Autodesk Inventor part; units mm, degrees
(part 8 of 9)
sketch "Sketch44" plane through (0, 0, 0) normal (1, 0, 0) x (0, 0, -1)
  arc A0 (-103.9823, -66.1369) -> (-104.5644, -66.2812) centre (-76.4174, -178.6042) ccw
  arc A1 (-99.4294, -84.7133) -> (-103.9823, -66.1369) centre (-101.7058, -75.4251) ccw
  arc A2 (-99.4294, -84.7133) -> (-99.9153, -84.8337) centre (-76.4174, -178.6042) ccw
  arc A3 (-104.5644, -66.2812) -> (-99.9153, -84.8337) centre (-102.2399, -75.5574) ccw
  arc A4 (-82.1853, 16.259) -> (-85.3603, 13.084) centre (-82.1853, 13.084) ccw
  line L0 (-85.3603, 13.084) -> (-85.3603, 6.734)
  arc A5 (-90.1228, 1.9715) -> (-85.3603, 6.734) centre (-90.1228, 6.734) ccw
  line L1 (-90.1228, 1.9715) -> (-121.8728, 1.9715)
  arc A6 (-126.6353, 6.734) -> (-121.8728, 1.9715) centre (-121.8728, 6.734) ccw
  line L2 (-126.6353, 6.734) -> (-126.6353, 13.084)
  arc A7 (-126.6353, 13.084) -> (-129.8103, 16.259) centre (-129.8103, 13.084) ccw
  line L3 (-129.8103, 16.259) -> (-132.3503, 16.259)
  arc A8 (-132.3503, 22.609) -> (-132.3503, 16.259) centre (-132.3503, 19.434) ccw
  line L4 (-132.3503, 22.609) -> (-129.8103, 22.609)
  arc A9 (-129.8103, 22.609) -> (-126.6353, 25.784) centre (-129.8103, 25.784) ccw
  line L5 (-126.6353, 25.784) -> (-126.6353, 32.134)
  arc A10 (-121.8728, 36.8965) -> (-126.6353, 32.134) centre (-121.8728, 32.134) ccw
  line L6 (-121.8728, 36.8965) -> (-90.1228, 36.8965)
  arc A11 (-85.3603, 32.134) -> (-90.1228, 36.8965) centre (-90.1228, 32.134) ccw
  line L7 (-85.3603, 32.134) -> (-85.3603, 25.784)
  arc A12 (-85.3603, 25.784) -> (-82.1853, 22.609) centre (-82.1853, 25.784) ccw
  line L8 (-82.1853, 22.609) -> (-79.6453, 22.609)
  arc A13 (-79.6453, 16.259) -> (-79.6453, 22.609) centre (-79.6453, 19.434) ccw
  line L9 (-79.6453, 16.259) -> (-82.1853, 16.259)
  line L10 (-112.3478, -13.7765) -> (-99.6478, -13.7765)
  arc A14 (-99.6478, -18.8819) -> (-99.6478, -13.7765) centre (-99.6478, -16.3292) ccw
  line L11 (-99.6478, -18.8819) -> (-112.3478, -18.8819)
  arc A15 (-112.3478, -13.7765) -> (-112.3478, -18.8819) centre (-112.3478, -16.3292) ccw
  circle A16 centre (-58.8554, 19.434) radius 2.4892
  line L12 (-177.4857, -133.2108) -> (-177.0061, -133.3781)
  arc A17 (-183.3071, -151.4366) -> (-177.0061, -133.3781) centre (-180.1566, -142.4074) ccw
  line L13 (-183.3071, -151.4366) -> (-183.7867, -151.2692)
  arc A18 (-177.4857, -133.2108) -> (-183.7867, -151.2692) centre (-180.6362, -142.24) ccw
  circle A19 centre (-76.4174, -178.6042) radius 13.335
  circle A20 centre (-187.1176, -166.8269) radius 2.4892
  circle A21 centre (-174.2102, -166.8866) radius 2.4892
  circle A22 centre (-167.2175, -120.5501) radius 2.4892
  circle A23 centre (-180.1195, -116.9252) radius 2.4892
  circle A24 centre (-193.0957, -120.1058) radius 2.4892
  circle A25 centre (-186.8225, -117.6771) radius 2.4892
  circle A26 centre (-173.4354, -117.9041) radius 2.4892
  circle A27 centre (-168.1768, -164.3742) radius 2.4892
  circle A28 centre (-180.6733, -167.7222) radius 2.4892
  circle A29 centre (-193.0957, -164.2646) radius 2.4892
  circle A30 centre (-85.7798, -94.9817) radius 2.4892
  circle A31 centre (-110.3931, -99.2933) radius 2.4892
  circle A32 centre (-101.8395, -50.0579) radius 2.4892
  circle A33 centre (-124.2369, -62.8574) radius 2.4892
  circle A34 centre (-110.6604, -51.6228) radius 2.4892
  circle A35 centre (-93.2858, -99.3592) radius 2.4892
  circle A36 centre (-118.4334, -56.0666) radius 2.4892
  circle A37 centre (-93.0185, -51.5569) radius 2.4892
  circle A38 centre (-101.8395, -100.8579) radius 2.4892
  circle A39 centre (-80.2428, -88.2574) radius 2.4892
  circle A40 centre (239.2356, -31.496) radius 3.3782
  circle A41 centre (223.7295, 90.3926) radius 3.3782
  circle A42 centre (239.2356, 31.496) radius 3.3782
  circle A43 centre (192.7107, -145.218) radius 3.3782
  line L14 (149.831, -89.2272) -> (89.9434, -38.9755)
  arc A44 (88.9, -36.7379) -> (89.9434, -38.9755) centre (91.821, -36.7379) ccw
  line L15 (88.9, -36.7379) -> (88.9, -15.621)
  arc A45 (91.821, -12.7) -> (88.9, -15.621) centre (91.821, -15.621) ccw
  line L16 (91.821, -12.7) -> (174.1799, -12.7)
  arc A46 (177.0893, -15.8819) -> (174.1799, -12.7) centre (174.1799, -15.621) ccw
  arc A47 (154.2425, -88.4425) -> (177.0893, -15.8819) centre (0, 0) ccw
  arc A48 (149.831, -89.2272) -> (154.2425, -88.4425) centre (151.7086, -86.9895) ccw
  line L17 (88.9, -0.254) -> (88.9, 0.254)
  arc A49 (91.821, 3.175) -> (88.9, 0.254) centre (91.821, 0.254) ccw
  line L18 (91.821, 3.175) -> (174.4218, 3.175)
  arc A50 (177.3428, 0.254) -> (174.4218, 3.175) centre (174.4218, 0.254) ccw
  line L19 (177.3428, 0.254) -> (177.3428, -0.254)
  arc A51 (174.4218, -3.175) -> (177.3428, -0.254) centre (174.4218, -0.254) ccw
  line L20 (174.4218, -3.175) -> (91.821, -3.175)
  arc A52 (88.9, -0.254) -> (91.821, -3.175) centre (91.821, -0.254) ccw
  arc A53 (177.0893, 15.8819) -> (169.6939, 53.0738) centre (0, 0) ccw
  arc A54 (174.1799, 12.7) -> (177.0893, 15.8819) centre (174.1799, 15.621) ccw
  line L21 (174.1799, 12.7) -> (91.821, 12.7)
  arc A55 (88.9, 15.621) -> (91.821, 12.7) centre (91.821, 15.621) ccw
  line L22 (88.9, 15.621) -> (88.9, 17.1891)
  arc A56 (90.5865, 19.8364) -> (88.9, 17.1891) centre (91.821, 17.1891) ccw
  line L23 (90.5865, 19.8364) -> (165.6716, 54.8492)
  arc A57 (169.6939, 53.0738) -> (165.6716, 54.8492) centre (166.9061, 52.2019) ccw
  arc A58 (180.8991, -105.7674) -> (203.0448, 51.8076) centre (0, 0) ccw
  arc A59 (204.8485, 54.889) -> (203.0448, 51.8076) centre (205.5059, 52.4355) ccw
  line L24 (204.8485, 54.889) -> (206.0753, 55.2177)
  arc A60 (209.1938, 53.3924) -> (206.0753, 55.2177) centre (206.7327, 52.7643) ccw
  arc A61 (186.3731, -108.9857) -> (209.1938, 53.3924) centre (0, 0) ccw
  arc A62 (182.8723, -109.8807) -> (186.3731, -108.9857) centre (184.1805, -107.7035) ccw
  line L25 (182.8723, -109.8807) -> (181.7836, -109.2266)
  arc A63 (180.8991, -105.7674) -> (181.7836, -109.2266) centre (183.0918, -107.0494) ccw
  arc A64 (159.1231, -92.6879) -> (178.5072, 45.237) centre (0, 0) ccw
  arc A65 (180.312, 48.3145) -> (178.5072, 45.237) centre (180.9694, 45.861) ccw
  line L26 (180.312, 48.3145) -> (181.5388, 48.6432)
  arc A66 (184.6584, 46.8139) -> (181.5388, 48.6432) centre (182.1962, 46.1897) ccw
  arc A67 (164.6013, -95.8992) -> (184.6584, 46.8139) centre (0, 0) ccw
  arc A68 (161.0985, -96.7977) -> (164.6013, -95.8992) centre (162.4067, -94.6205) ccw
  line L27 (161.0985, -96.7977) -> (160.0098, -96.1436)
  arc A69 (159.1231, -92.6879) -> (160.0098, -96.1436) centre (161.3179, -93.9664) ccw
  line L28 (171.9854, -103.3393) -> (170.8967, -102.6851)
  arc A70 (170.0112, -99.2275) -> (170.8967, -102.6851) centre (172.2049, -100.5079) ccw
  arc A71 (170.0112, -99.2275) -> (190.7761, 48.5222) centre (0, 0) ccw
  arc A72 (192.5803, 51.6017) -> (190.7761, 48.5222) centre (193.2377, 49.1483) ccw
  line L29 (192.5803, 51.6017) -> (193.8071, 51.9305)
  arc A73 (196.9261, 50.1033) -> (193.8071, 51.9305) centre (194.4645, 49.477) ccw
  arc A74 (175.4872, -102.4426) -> (196.9261, 50.1033) centre (0, 0) ccw
  arc A75 (171.9854, -103.3393) -> (175.4872, -102.4426) centre (173.2936, -101.1621) ccw
  circle A76 centre (187.962, 68.4126) radius 2.5527
  circle A77 centre (0, 0) radius 13.335
  circle A78 centre (160.7915, -118.9794) radius 2.5527
  circle A79 centre (145.0649, -113.4346) radius 2.5527
  circle A80 centre (122.2368, -242.899) radius 2.5527
  circle A81 centre (70.3186, -242.899) radius 2.5527
  circle A82 centre (97.9437, -242.899) radius 2.5527
  circle A83 centre (145.0649, -242.899) radius 2.5527
  circle A84 centre (-116.932, -242.899) radius 2.5527
  circle A85 centre (-116.932, -179.399) radius 2.5527
  circle A86 centre (-148.682, -179.399) radius 2.5527
  circle A87 centre (-186.782, -39.699) radius 2.5527
  circle A88 centre (-186.782, -242.899) radius 2.5527
  circle A89 centre (67.218, 63.5) radius 2.5527
  circle A90 centre (-59.782, 63.5) radius 2.5527
  circle A91 centre (-8.982, 63.5) radius 2.5527
  circle A92 centre (143.418, 63.5) radius 2.5527
  circle A93 centre (-186.782, -179.399) radius 2.5527
  circle A94 centre (-148.682, -39.699) radius 2.5527
  circle A95 centre (-116.932, -39.699) radius 2.5527
  circle A96 centre (-148.682, -242.899) radius 2.5527
  circle A97 centre (11.1125, -19.2474) radius 2.2479
  circle A98 centre (-22.225, 0) radius 2.2479
  circle A99 centre (11.1125, 19.2474) radius 2.2479
  circle A100 centre (22.225, 0) radius 2.2479
  circle A101 centre (-11.1125, 19.2474) radius 2.2479
  circle A102 centre (-11.1125, -19.2474) radius 2.2479
  line L30 (-80.5978, 54.7781) -> (-131.3978, 54.7781)
  arc A103 (-131.3978, 59.8835) -> (-131.3978, 54.7781) centre (-131.3978, 57.3308) ccw
  line L31 (-131.3978, 59.8835) -> (-80.5978, 59.8835)
  arc A104 (-80.5978, 54.7781) -> (-80.5978, 59.8835) centre (-80.5978, 57.3308) ccw
  circle A105 centre (-123.52, 44.45) radius 2.4892
  arc A106 (-166.8187, -7.1514) -> (-170.0188, -10.965) centre (-168.4187, -9.0582) ccw
  arc A107 (-166.8187, -7.1514) -> (-135.2171, -21.8874) centre (-123.52, 44.45) ccw
  arc A108 (-136.0816, -26.7902) -> (-135.2171, -21.8874) centre (-135.6494, -24.3388) ccw
  arc A109 (-170.0188, -10.965) -> (-136.0816, -26.7902) centre (-123.52, 44.45) ccw
  arc A110 (-196.307, 76.2) -> (-199.482, 73.025) centre (-196.307, 73.025) ccw
  line L32 (-199.482, 73.025) -> (-199.482, -252.424)
  arc A111 (-199.482, -252.424) -> (-196.307, -255.599) centre (-196.307, -252.424) ccw
  line L33 (-196.307, -255.599) -> (147.8383, -255.599)
  arc A112 (147.8383, -255.599) -> (150.6952, -253.8092) centre (147.8383, -252.424) ccw
  line L34 (194.4526, -163.563) -> (150.6952, -253.8092)
  arc A113 (194.8736, -162.9119) -> (194.4526, -163.563) centre (197.3095, -164.9483) ccw
  arc A114 (194.8736, -162.9119) -> (235.5329, 95.0804) centre (0, 0) ccw
  arc A115 (235.5329, 95.0804) -> (218.389, 101.8364) centre (223.7562, 90.3263) ccw
  line L35 (218.389, 101.8364) -> (173.6183, 80.9596)
  arc A116 (152.1493, 76.2) -> (173.6183, 80.9596) centre (152.1493, 127) ccw
  line L36 (152.1493, 76.2) -> (-196.307, 76.2)
  arc A117 (-85.6539, -48.4094) -> (-88.99, -46.6745) centre (-90.1204, -52.923) ccw
  arc A118 (-114.689, -104.2414) -> (-85.6539, -48.4094) centre (-101.8395, -75.4579) ccw
  arc A119 (-118.0252, -102.5065) -> (-114.689, -104.2414) centre (-113.5587, -97.9928) ccw
  arc A120 (-88.99, -46.6745) -> (-118.0252, -102.5065) centre (-101.8395, -75.4579) ccw
  arc A121 (-84.1306, -35.1868) -> (-84.8012, -35.3982) centre (-84.3454, -35.6751) ccw
  arc A122 (-85.259, -35.965) -> (-84.8012, -35.3982) centre (-87.1419, -33.9761) ccw
  arc A123 (-87.6678, -35.0381) -> (-85.259, -35.965) centre (-86.2421, -34.9266) ccw
  arc A124 (-87.6275, -34.3106) -> (-87.6678, -35.0381) centre (-84.9373, -34.8245) ccw
  arc A125 (-87.6275, -34.3106) -> (-87.9834, -33.7042) centre (-88.1514, -34.2105) ccw
  arc A126 (-87.9834, -33.7042) -> (-88.7509, -33.4573) centre (-101.8395, -75.4579) ccw
  arc A127 (-88.7509, -33.4573) -> (-89.3936, -33.7424) centre (-88.9096, -33.9665) ccw
  arc A128 (-89.7851, -34.3569) -> (-89.3936, -33.7424) centre (-91.8788, -32.5913) ccw
  arc A129 (-92.2825, -33.7055) -> (-89.7851, -34.3569) centre (-90.8783, -33.4351) ccw
  arc A130 (-92.3239, -32.978) -> (-92.2825, -33.7055) centre (-89.5931, -33.1875) ccw
  arc A131 (-92.3239, -32.978) -> (-92.7455, -32.4154) centre (-92.8557, -32.9372) ccw
  arc A132 (-92.7455, -32.4154) -> (-93.5358, -32.2559) centre (-101.8395, -75.4579) ccw
  arc A133 (-93.5358, -32.2559) -> (-94.1425, -32.6112) centre (-93.6365, -32.7797) ccw
  arc A134 (-94.4627, -33.2657) -> (-94.1425, -32.6112) centre (-96.741, -31.7456) ccw
  arc A135 (-97.0174, -32.898) -> (-94.4627, -33.2657) centre (-95.6523, -32.472) ccw
  arc A136 (-97.14, -32.1797) -> (-97.0174, -32.898) centre (-94.4029, -32.0822) ccw
  arc A137 (-97.14, -32.1797) -> (-97.6219, -31.6678) centre (-97.673, -32.1987) ccw
  arc A138 (-97.6219, -31.6678) -> (-98.4251, -31.5978) centre (-101.8395, -75.4579) ccw
  arc A139 (-98.4251, -31.5978) -> (-98.9883, -32.0188) centre (-98.4665, -32.1296) ccw
  arc A140 (-99.2331, -32.7051) -> (-98.9883, -32.0188) centre (-101.6673, -31.4496) ccw
  arc A141 (-101.8129, -32.6257) -> (-99.2331, -32.7051) centre (-100.5041, -32.0496) ccw
  arc A142 (-102.0151, -31.9257) -> (-101.8129, -32.6257) centre (-99.3062, -31.5223) ccw
  arc A143 (-102.0151, -31.9257) -> (-102.5514, -31.4709) centre (-102.5427, -32.0042) ccw
  arc A144 (-102.5514, -31.4709) -> (-103.3573, -31.4913) centre (-101.8395, -75.4579) ccw
  arc A145 (-103.3573, -31.4913) -> (-103.8698, -31.9727) centre (-103.3389, -32.0244) ccw
  arc A146 (-104.0363, -32.6821) -> (-103.8698, -31.9727) centre (-106.5957, -31.7071) ccw
  arc A147 (-106.6088, -32.892) -> (-104.0363, -32.6821) centre (-105.3727, -32.173) ccw
  arc A148 (-106.8881, -32.2191) -> (-106.6088, -32.892) centre (-104.2414, -31.5149) ccw
  arc A149 (-106.8881, -32.2191) -> (-107.4719, -31.8272) centre (-107.4036, -32.3562) ccw
  arc A150 (-107.4719, -31.8272) -> (-108.2705, -31.9377) centre (-101.8395, -75.4579) ccw
  arc A151 (-108.2705, -31.9377) -> (-108.7259, -32.4734) centre (-108.1925, -32.4654) ccw
  arc A152 (-108.8119, -33.197) -> (-108.7259, -32.4734) centre (-111.4644, -32.5147) ccw
  arc A153 (-111.3446, -33.6937) -> (-108.8119, -33.197) centre (-110.1968, -32.8407) ccw
  arc A154 (-111.6976, -33.0562) -> (-111.3446, -33.6937) centre (-109.1463, -32.0601) ccw
  arc A155 (-111.6976, -33.0562) -> (-112.3216, -32.7321) centre (-112.1945, -33.2502) ccw
  arc A156 (-112.3216, -32.7321) -> (-113.1028, -32.9314) centre (-101.8395, -75.4579) ccw
  arc A157 (-113.1028, -32.9314) -> (-113.4953, -33.5147) centre (-112.9662, -33.447) ccw
  arc A158 (-113.4998, -34.2434) -> (-113.4953, -33.5147) centre (-116.212, -33.8623) ccw
  arc A159 (-115.961, -35.0205) -> (-113.4998, -34.2434) centre (-114.9159, -34.0444) ccw
  arc A160 (-116.3831, -34.4266) -> (-115.961, -35.0205) centre (-113.9594, -33.1511) ccw
  arc A161 (-116.3831, -34.4266) -> (-117.0394, -34.1744) centre (-116.8551, -34.675) ccw
  arc A162 (-117.0394, -34.1744) -> (-117.7934, -34.4599) centre (-101.8395, -75.4579) ccw
  arc A163 (-117.7934, -34.4599) -> (-118.1182, -35.0835) centre (-117.6, -34.957) ccw
  arc A164 (-118.041, -35.8081) -> (-118.1182, -35.0835) centre (-120.7788, -35.7331) ccw
  arc A165 (-120.3998, -36.8559) -> (-118.041, -35.8081) centre (-119.4705, -35.7689) ccw
  arc A166 (-120.8857, -36.3129) -> (-120.3998, -36.8559) centre (-118.6201, -34.7741) ccw
  arc A167 (-120.8857, -36.3129) -> (-121.5661, -36.1358) centre (-121.327, -36.6126) ccw
  arc A168 (-121.5661, -36.1358) -> (-122.2834, -36.5039) centre (-101.8395, -75.4579) ccw
  arc A169 (-122.2834, -36.5039) -> (-122.5363, -37.16) centre (-122.0356, -36.9763) ccw
  arc A170 (-122.3785, -37.8714) -> (-122.5363, -37.16) centre (-125.1075, -38.1034) ccw
  arc A171 (-124.6051, -39.1767) -> (-122.3785, -37.8714) centre (-123.8034, -37.9925) ccw
  arc A172 (-125.1488, -38.6915) -> (-124.6051, -39.1767) centre (-123.0697, -36.9087) ccw
  arc A173 (-125.1488, -38.6915) -> (-125.8448, -38.5918) centre (-125.5537, -39.0388) ccw
  arc A174 (-125.8448, -38.5918) -> (-126.5163, -39.0379) centre (-101.8395, -75.4579) ccw
  arc A175 (-126.5163, -39.0379) -> (-126.6942, -39.7181) centre (-126.2171, -39.4795) ccw
  arc A176 (-126.4578, -40.4073) -> (-126.6942, -39.7181) centre (-129.1436, -40.9435) ccw
  arc A177 (-128.5242, -41.9537) -> (-126.4578, -40.4073) centre (-127.8601, -40.6873) ccw
  arc A178 (-129.1188, -41.5325) -> (-128.5242, -41.9537) centre (-127.2523, -39.5281) ccw
  arc A179 (-129.1188, -41.5325) -> (-129.8215, -41.5113) centre (-129.4823, -41.9229) ccw
  arc A180 (-129.8215, -41.5113) -> (-130.4389, -42.0298) centre (-101.8395, -75.4579) ccw
  arc A181 (-130.4389, -42.0298) -> (-130.5395, -42.7257) centre (-130.0922, -42.4351) ccw
  arc A182 (-130.2274, -43.3841) -> (-130.5395, -42.7257) centre (-132.8363, -44.2176) ccw
  arc A183 (-132.1077, -45.1521) -> (-130.2274, -43.3841) centre (-131.5896, -43.8193) ccw
  arc A184 (-132.7457, -44.8002) -> (-132.1077, -45.1521) centre (-131.1154, -42.5994) ccw
  arc A185 (-132.7457, -44.8002) -> (-133.4464, -44.8577) centre (-133.0632, -45.2288) ccw
  arc A186 (-133.4464, -44.8577) -> (-134.0019, -45.4421) centre (-101.8395, -75.4579) ccw
  arc A187 (-134.0019, -45.4421) -> (-134.0239, -46.1449) centre (-133.6119, -45.806) ccw
  arc A188 (-133.64, -46.7642) -> (-134.0239, -46.1449) centre (-136.1392, -47.8845) ccw
  arc A189 (-135.3105, -48.7317) -> (-133.64, -46.7642) centre (-134.9449, -47.3492) ccw
  arc A190 (-135.9839, -48.4533) -> (-135.3105, -48.7317) centre (-134.6103, -46.0839) ccw
  arc A191 (-135.9839, -48.4533) -> (-136.6738, -48.589) centre (-136.2514, -48.9148) ccw
  arc A192 (-136.6738, -48.589) -> (-137.1604, -49.2319) centre (-101.8395, -75.4579) ccw
  arc A193 (-137.1604, -49.2319) -> (-137.1035, -49.9327) centre (-136.7321, -49.5499) ccw
  arc A194 (-136.6528, -50.5051) -> (-137.1035, -49.9327) centre (-139.0108, -51.8983) ccw
  arc A195 (-138.0925, -52.6473) -> (-136.6528, -50.5051) centre (-137.884, -51.2325) ccw
  arc A196 (-138.7928, -52.4461) -> (-138.0925, -52.6473) centre (-137.6931, -49.9377) ccw
  arc A197 (-138.7928, -52.4461) -> (-139.4631, -52.6581) centre (-139.007, -52.9346) ccw
  arc A198 (-139.4631, -52.6581) -> (-139.8746, -53.3515) centre (-101.8395, -75.4579) ccw
  arc A199 (-139.8746, -53.3515) -> (-139.7397, -54.0415) centre (-139.4135, -53.6195) ccw
  arc A200 (-139.2277, -54.5599) -> (-139.7397, -54.0415) centre (-141.4149, -56.2083) ccw
  arc A201 (-140.4185, -56.8497) -> (-139.2277, -54.5599) centre (-140.3697, -55.4205) ccw
  arc A202 (-141.137, -56.7282) -> (-140.4185, -56.8497) centre (-140.325, -54.1125) ccw
  arc A203 (-141.137, -56.7282) -> (-141.7793, -57.014) centre (-141.2951, -57.2376) ccw
  arc A204 (-141.7793, -57.014) -> (-142.1106, -57.749) centre (-101.8395, -75.4579) ccw
  arc A205 (-142.1106, -57.749) -> (-141.8993, -58.4196) centre (-141.6224, -57.9638) ccw
  arc A206 (-141.3324, -58.8774) -> (-141.8993, -58.4196) centre (-143.3214, -60.7603) ccw
  arc A207 (-142.2594, -61.2862) -> (-141.3324, -58.8774) centre (-142.3709, -59.8605) ccw
  arc A208 (-142.9869, -61.2459) -> (-142.2594, -61.2862) centre (-142.473, -58.5557) ccw
  arc A209 (-142.9869, -61.2459) -> (-143.5933, -61.6018) centre (-143.087, -61.7698) ccw
  arc A210 (-143.5933, -61.6018) -> (-143.8402, -62.3693) centre (-101.8395, -75.4579) ccw
  arc A211 (-143.8402, -62.3693) -> (-143.5551, -63.012) centre (-143.3309, -62.528) ccw
  arc A212 (-142.9405, -63.4035) -> (-143.5551, -63.012) centre (-144.7061, -65.4972) ccw
  arc A213 (-143.592, -65.9009) -> (-142.9405, -63.4035) centre (-143.8624, -64.4967) ccw
  arc A214 (-144.3194, -65.9423) -> (-143.592, -65.9009) centre (-144.1099, -63.2115) ccw
  arc A215 (-144.3194, -65.9423) -> (-144.8821, -66.3639) centre (-144.3602, -66.4741) ccw
  arc A216 (-144.8821, -66.3639) -> (-145.0416, -67.1542) centre (-101.8395, -75.4579) ccw
  arc A217 (-145.0416, -67.1542) -> (-144.6863, -67.7609) centre (-144.5177, -67.2549) ccw
  arc A218 (-144.0318, -68.0811) -> (-144.6863, -67.7609) centre (-145.5519, -70.3594) ccw
  arc A219 (-144.3995, -70.6358) -> (-144.0318, -68.0811) centre (-144.8255, -69.2707) ccw
  arc A220 (-145.1178, -70.7584) -> (-144.3995, -70.6358) centre (-145.2153, -68.0213) ccw
  arc A221 (-145.1178, -70.7584) -> (-145.6297, -71.2403) centre (-145.0988, -71.2914) ccw
  arc A222 (-145.6297, -71.2403) -> (-145.6996, -72.0435) centre (-101.8395, -75.4579) ccw
  arc A223 (-145.6996, -72.0435) -> (-145.2787, -72.6067) centre (-145.1678, -72.0849) ccw
  arc A224 (-144.5924, -72.8515) -> (-145.2787, -72.6067) centre (-145.8479, -75.2857) ccw
  arc A225 (-144.6718, -75.4313) -> (-144.5924, -72.8515) centre (-145.2479, -74.1225) ccw
  arc A226 (-145.3718, -75.6336) -> (-144.6718, -75.4313) centre (-145.7752, -72.9246) ccw
  arc A227 (-145.3718, -75.6336) -> (-145.8266, -76.1698) centre (-145.2932, -76.1611) ccw
  arc A228 (-145.8266, -76.1698) -> (-145.8061, -76.9757) centre (-101.8395, -75.4579) ccw
  arc A229 (-145.8061, -76.9757) -> (-145.3248, -77.4882) centre (-145.2731, -76.9573) ccw
  arc A230 (-144.6154, -77.6547) -> (-145.3248, -77.4882) centre (-145.5904, -80.2141) ccw
  arc A231 (-144.4054, -80.2272) -> (-144.6154, -77.6547) centre (-145.1245, -78.9911) ccw
  arc A232 (-145.0784, -80.5065) -> (-144.4054, -80.2272) centre (-145.7826, -77.8598) ccw
  arc A233 (-145.0784, -80.5065) -> (-145.4703, -81.0903) centre (-144.9413, -81.022) ccw
  arc A234 (-145.4703, -81.0903) -> (-145.3598, -81.8889) centre (-101.8395, -75.4579) ccw
  arc A235 (-145.3598, -81.8889) -> (-144.824, -82.3443) centre (-144.8321, -81.8109) ccw
  arc A236 (-144.1005, -82.4303) -> (-144.824, -82.3443) centre (-144.7828, -85.0828) ccw
  arc A237 (-143.6038, -84.9631) -> (-144.1005, -82.4303) centre (-144.4567, -83.8152) ccw
  arc A238 (-144.2413, -85.316) -> (-143.6038, -84.9631) centre (-145.2374, -82.7647) ccw
  arc A239 (-144.2413, -85.316) -> (-144.5653, -85.94) centre (-144.0473, -85.8129) ccw
  arc A240 (-144.5653, -85.94) -> (-144.3661, -86.7212) centre (-101.8395, -75.4579) ccw
  arc A241 (-144.3661, -86.7212) -> (-143.7827, -87.1137) centre (-143.8504, -86.5846) ccw
  arc A242 (-143.0541, -87.1182) -> (-143.7827, -87.1137) centre (-143.4351, -89.8304) ccw
  arc A243 (-142.277, -89.5794) -> (-143.0541, -87.1182) centre (-143.2531, -88.5343) ccw
  arc A244 (-142.8709, -90.0015) -> (-142.277, -89.5794) centre (-144.1464, -87.5778) ccw
  arc A245 (-142.8709, -90.0015) -> (-143.1231, -90.6578) centre (-142.6225, -90.4735) ccw
  arc A246 (-143.1231, -90.6578) -> (-142.8376, -91.4118) centre (-101.8395, -75.4579) ccw
  arc A247 (-142.8376, -91.4118) -> (-142.214, -91.7366) centre (-142.3405, -91.2184) ccw
  arc A248 (-141.4894, -91.6594) -> (-142.214, -91.7366) centre (-141.5644, -94.3972) ccw
  arc A249 (-140.4416, -94.0182) -> (-141.4894, -91.6594) centre (-141.5286, -93.0889) ccw
  arc A250 (-140.9846, -94.5041) -> (-140.4416, -94.0182) centre (-142.5234, -92.2385) ccw
  arc A251 (-140.9846, -94.5041) -> (-141.1616, -95.1845) centre (-140.6849, -94.9454) ccw
  arc A252 (-141.1616, -95.1845) -> (-140.7935, -95.9018) centre (-101.8395, -75.4579) ccw
  arc A253 (-140.7935, -95.9018) -> (-140.1375, -96.1547) centre (-140.3212, -95.654) ccw
  arc A254 (-139.4261, -95.997) -> (-140.1375, -96.1547) centre (-139.1941, -98.7259) ccw
  arc A255 (-138.1208, -98.2235) -> (-139.4261, -95.997) centre (-139.305, -97.4218) ccw
  arc A256 (-138.6059, -98.7672) -> (-138.1208, -98.2235) centre (-140.3888, -96.6881) ccw
  arc A257 (-138.6059, -98.7672) -> (-138.7057, -99.4632) centre (-138.2587, -99.1721) ccw
  arc A258 (-138.7057, -99.4632) -> (-138.2596, -100.1348) centre (-101.8395, -75.4579) ccw
  arc A259 (-138.2596, -100.1348) -> (-137.5794, -100.3126) centre (-137.818, -99.8356) ccw
  arc A260 (-136.8901, -100.0762) -> (-137.5794, -100.3126) centre (-136.354, -102.762) ccw
  arc A261 (-135.3437, -102.1426) -> (-136.8901, -100.0762) centre (-136.6102, -101.4785) ccw
  arc A262 (-135.7649, -102.7372) -> (-135.3437, -102.1426) centre (-137.7693, -100.8707) ccw
  arc A263 (-135.7649, -102.7372) -> (-135.7862, -103.4399) centre (-135.3746, -103.1007) ccw
  arc A264 (-135.7862, -103.4399) -> (-135.2677, -104.0573) centre (-101.8395, -75.4579) ccw
  arc A265 (-135.2677, -104.0573) -> (-134.5718, -104.1579) centre (-134.8624, -103.7106) ccw
  arc A266 (-133.9134, -103.8458) -> (-134.5718, -104.1579) centre (-133.0799, -106.4547) ccw
  arc A267 (-132.1453, -105.7261) -> (-133.9134, -103.8458) centre (-133.4782, -105.208) ccw
  arc A268 (-132.4973, -106.3641) -> (-132.1453, -105.7261) centre (-134.6981, -104.7338) ccw
  arc A269 (-132.4973, -106.3641) -> (-132.4397, -107.0648) centre (-132.0687, -106.6816) ccw
  arc A270 (-132.4397, -107.0648) -> (-131.8554, -107.6203) centre (-101.8395, -75.4579) ccw
  arc A271 (-131.8554, -107.6203) -> (-131.1526, -107.6423) centre (-131.4914, -107.2303) ccw
  arc A272 (-130.5333, -107.2584) -> (-131.1526, -107.6423) centre (-129.4129, -109.7576) ccw
  arc A273 (-128.5658, -108.9289) -> (-130.5333, -107.2584) centre (-129.9483, -108.5633) ccw
  arc A274 (-128.8442, -109.6023) -> (-128.5658, -108.9289) centre (-131.2136, -108.2287) ccw
  arc A275 (-128.8442, -109.6023) -> (-128.7085, -110.2922) centre (-128.3827, -109.8699) ccw
  arc A276 (-128.7085, -110.2922) -> (-128.0656, -110.7788) centre (-101.8395, -75.4579) ccw
  arc A277 (-128.0656, -110.7788) -> (-127.3648, -110.722) centre (-127.7476, -110.3505) ccw
  arc A278 (-126.7923, -110.2712) -> (-127.3648, -110.722) centre (-125.3992, -112.6292) ccw
  arc A279 (-124.6502, -111.7109) -> (-126.7923, -110.2712) centre (-126.065, -111.5024) ccw
  arc A280 (-124.8514, -112.4112) -> (-124.6502, -111.7109) centre (-127.3598, -111.3115) ccw
  arc A281 (-124.8514, -112.4112) -> (-124.6393, -113.0815) centre (-124.3629, -112.6254) ccw
  arc A282 (-124.6393, -113.0815) -> (-123.946, -113.4931) centre (-101.8395, -75.4579) ccw
  arc A283 (-123.946, -113.4931) -> (-123.256, -113.3581) centre (-123.678, -113.0319) ccw
  arc A284 (-122.7376, -112.8461) -> (-123.256, -113.3581) centre (-121.0892, -115.0333) ccw
  arc A285 (-120.4477, -114.0369) -> (-122.7376, -112.8461) centre (-121.8769, -113.9881) ccw
  arc A286 (-120.5693, -114.7554) -> (-120.4477, -114.0369) centre (-123.185, -113.9434) ccw
  arc A287 (-120.5693, -114.7554) -> (-120.2835, -115.3977) centre (-120.0598, -114.9135) ccw
  arc A288 (-120.2835, -115.3977) -> (-119.5484, -115.729) centre (-101.8395, -75.4579) ccw
  arc A289 (-119.5484, -115.729) -> (-118.8779, -115.5177) centre (-119.3337, -115.2408) ccw
  arc A290 (-118.4201, -114.9508) -> (-118.8779, -115.5177) centre (-116.5372, -116.9398) ccw
  arc A291 (-116.0113, -115.8778) -> (-118.4201, -114.9508) centre (-117.4369, -115.9893) ccw
  arc A292 (-116.0516, -116.6053) -> (-116.0113, -115.8778) centre (-118.7417, -116.0914) ccw
  arc A293 (-116.0516, -116.6053) -> (-115.6957, -117.2117) centre (-115.5277, -116.7054) ccw
  arc A294 (-115.6957, -117.2117) -> (-114.9282, -117.4586) centre (-101.8395, -75.4579) ccw
  arc A295 (-114.9282, -117.4586) -> (-114.2855, -117.1735) centre (-114.7695, -116.9493) ccw
  arc A296 (-113.894, -116.5589) -> (-114.2855, -117.1735) centre (-111.8002, -118.3245) ccw
  arc A297 (-111.3966, -117.2104) -> (-113.894, -116.5589) centre (-112.8008, -117.4808) ccw
  arc A298 (-111.3552, -117.9379) -> (-111.3966, -117.2104) centre (-114.086, -117.7283) ccw
  arc A299 (-111.3552, -117.9379) -> (-110.9336, -118.5005) centre (-110.8233, -117.9787) ccw
  arc A300 (-110.9336, -118.5005) -> (-110.1433, -118.66) centre (-101.8395, -75.4579) ccw
  arc A301 (-110.1433, -118.66) -> (-109.5365, -118.3047) centre (-110.0426, -118.1361) ccw
  arc A302 (-109.2163, -117.6502) -> (-109.5365, -118.3047) centre (-106.9381, -119.1703) ccw
  arc A303 (-106.6617, -118.0179) -> (-109.2163, -117.6502) centre (-108.0268, -118.4439) ccw
  arc A304 (-106.5391, -118.7362) -> (-106.6617, -118.0179) centre (-109.2762, -118.8337) ccw
  arc A305 (-106.5391, -118.7362) -> (-106.0572, -119.2481) centre (-106.006, -118.7172) ccw
  arc A306 (-106.0572, -119.2481) -> (-105.254, -119.318) centre (-101.8395, -75.4579) ccw
  arc A307 (-105.254, -119.318) -> (-104.6908, -118.8971) centre (-105.2126, -118.7862) ccw
  arc A308 (-104.4459, -118.2108) -> (-104.6908, -118.8971) centre (-102.0118, -119.4663) ccw
  arc A309 (-101.8662, -118.2902) -> (-104.4459, -118.2108) centre (-103.175, -118.8663) ccw
  arc A310 (-101.6639, -118.9902) -> (-101.8662, -118.2902) centre (-104.3729, -119.3936) ccw
  arc A311 (-101.6639, -118.9902) -> (-101.1277, -119.445) centre (-101.1363, -118.9117) ccw
  arc A312 (-101.1277, -119.445) -> (-100.3217, -119.4246) centre (-101.8395, -75.4579) ccw
  arc A313 (-100.3217, -119.4246) -> (-99.8092, -118.9432) centre (-100.3401, -118.8915) ccw
  arc A314 (-99.6427, -118.2338) -> (-99.8092, -118.9432) centre (-97.0833, -119.2088) ccw
  arc A315 (-97.0703, -118.0239) -> (-99.6427, -118.2338) centre (-98.3064, -118.7429) ccw
  arc A316 (-96.791, -118.6968) -> (-97.0703, -118.0239) centre (-99.4377, -119.401) ccw
  arc A317 (-96.791, -118.6968) -> (-96.2072, -119.0887) centre (-96.2755, -118.5597) ccw
  arc A318 (-96.2072, -119.0887) -> (-95.4086, -118.9782) centre (-101.8395, -75.4579) ccw
  arc A319 (-95.4086, -118.9782) -> (-94.9532, -118.4425) centre (-95.4866, -118.4505) ccw
  arc A320 (-94.8672, -117.7189) -> (-94.9532, -118.4425) centre (-92.2147, -118.4012) ccw
  arc A321 (-92.3344, -117.2222) -> (-94.8672, -117.7189) centre (-93.4822, -118.0752) ccw
  arc A322 (-91.9815, -117.8597) -> (-92.3344, -117.2222) centre (-94.5328, -118.8558) ccw
  arc A323 (-91.9815, -117.8597) -> (-91.3575, -118.1837) centre (-91.4846, -117.6657) ccw
  arc A324 (-91.3575, -118.1837) -> (-90.5763, -117.9845) centre (-101.8395, -75.4579) ccw
  arc A325 (-90.5763, -117.9845) -> (-90.1838, -117.4012) centre (-90.7129, -117.4689) ccw
  arc A326 (-90.1793, -116.6725) -> (-90.1838, -117.4012) centre (-87.4671, -117.0535) ccw
  arc A327 (-87.7181, -115.8954) -> (-90.1793, -116.6725) centre (-88.7632, -116.8715) ccw
  arc A328 (-87.296, -116.4893) -> (-87.7181, -115.8954) centre (-89.7197, -117.7648) ccw
  arc A329 (-87.296, -116.4893) -> (-86.6397, -116.7415) centre (-86.824, -116.2409) ccw
  arc A330 (-86.6397, -116.7415) -> (-85.8857, -116.456) centre (-101.8395, -75.4579) ccw
  arc A331 (-85.8857, -116.456) -> (-85.5609, -115.8324) centre (-86.0791, -115.9589) ccw
  arc A332 (-85.638, -115.1078) -> (-85.5609, -115.8324) centre (-82.9002, -115.1828) ccw
  arc A333 (-83.2793, -114.06) -> (-85.638, -115.1078) centre (-84.2086, -115.147) ccw
  arc A334 (-82.7934, -114.603) -> (-83.2793, -114.06) centre (-85.059, -116.1418) ccw
  arc A335 (-82.7934, -114.603) -> (-82.1129, -114.78) centre (-82.3521, -114.3033) ccw
  arc A336 (-82.1129, -114.78) -> (-81.3956, -114.4119) centre (-101.8395, -75.4579) ccw
  arc A337 (-81.3956, -114.4119) -> (-81.1428, -113.7559) centre (-81.6435, -113.9396) ccw
  arc A338 (-81.3005, -113.0445) -> (-81.1428, -113.7559) centre (-78.5716, -112.8125) ccw
  arc A339 (-79.074, -111.7392) -> (-81.3005, -113.0445) centre (-79.8756, -112.9234) ccw
  arc A340 (-78.5303, -112.2243) -> (-79.074, -111.7392) centre (-80.6094, -114.0072) ccw
  arc A341 (-78.5303, -112.2243) -> (-77.8343, -112.3241) centre (-78.1254, -111.8771) ccw
  arc A342 (-77.8343, -112.3241) -> (-77.1627, -111.878) centre (-101.8395, -75.4579) ccw
  arc A343 (-77.1627, -111.878) -> (-76.9849, -111.1978) centre (-77.4619, -111.4364) ccw
  arc A344 (-77.2213, -110.5086) -> (-76.9849, -111.1978) centre (-74.5355, -109.9724) ccw
  arc A345 (-75.1549, -108.9621) -> (-77.2213, -110.5086) centre (-75.819, -110.2286) ccw
  arc A346 (-74.5603, -109.3834) -> (-75.1549, -108.9621) centre (-76.4267, -111.3877) ccw
  arc A347 (-74.5603, -109.3834) -> (-73.8575, -109.4046) centre (-74.1968, -108.993) ccw
  arc A348 (-73.8575, -109.4046) -> (-73.2401, -108.8861) centre (-101.8395, -75.4579) ccw
  arc A349 (-73.2401, -108.8861) -> (-73.1396, -108.1902) centre (-73.5869, -108.4808) ccw
  arc A350 (-73.4517, -107.5318) -> (-73.1396, -108.1902) centre (-70.8428, -106.6983) ccw
  arc A351 (-71.5714, -105.7637) -> (-73.4517, -107.5318) centre (-72.0895, -107.0966) ccw
  arc A352 (-70.9334, -106.1157) -> (-71.5714, -105.7637) centre (-72.5637, -108.3165) ccw
  arc A353 (-70.9334, -106.1157) -> (-70.2327, -106.0581) centre (-70.6159, -105.6871) ccw
  arc A354 (-70.2327, -106.0581) -> (-69.6772, -105.4738) centre (-101.8395, -75.4579) ccw
  arc A355 (-69.6772, -105.4738) -> (-69.6552, -104.771) centre (-70.0672, -105.1098) ccw
  arc A356 (-70.039, -104.1517) -> (-69.6552, -104.771) centre (-67.5398, -103.0314) ccw
  arc A357 (-68.3685, -102.1842) -> (-70.039, -104.1517) centre (-68.7341, -103.5667) ccw
  arc A358 (-67.6951, -102.4626) -> (-68.3685, -102.1842) centre (-69.0688, -104.832) ccw
  arc A359 (-67.6951, -102.4626) -> (-67.0053, -102.3269) centre (-67.4276, -102.0011) ccw
  arc A360 (-67.0053, -102.3269) -> (-66.5187, -101.684) centre (-101.8395, -75.4579) ccw
  arc A361 (-66.5187, -101.684) -> (-66.5755, -100.9832) centre (-66.947, -101.366) ccw
  arc A362 (-67.0263, -100.4107) -> (-66.5755, -100.9832) centre (-64.6683, -99.0176) ccw
  arc A363 (-65.5866, -98.2686) -> (-67.0263, -100.4107) centre (-65.7951, -99.6834) ccw
  arc A364 (-64.8863, -98.4698) -> (-65.5866, -98.2686) centre (-65.986, -100.9782) ccw
  arc A365 (-64.8863, -98.4698) -> (-64.2159, -98.2577) centre (-64.6721, -97.9813) ccw
  arc A366 (-64.2159, -98.2577) -> (-63.8044, -97.5644) centre (-101.8395, -75.4579) ccw
  arc A367 (-63.8044, -97.5644) -> (-63.9393, -96.8744) centre (-64.2656, -97.2964) ccw
  arc A368 (-64.4514, -96.356) -> (-63.9393, -96.8744) centre (-62.2642, -94.7076) ccw
  arc A369 (-63.2606, -94.0662) -> (-64.4514, -96.356) centre (-63.3094, -95.4953) ccw
  arc A370 (-62.5421, -94.1877) -> (-63.2606, -94.0662) centre (-63.354, -96.8034) ccw
  arc A371 (-62.5421, -94.1877) -> (-61.8997, -93.9019) centre (-62.384, -93.6782) ccw
  arc A372 (-61.8997, -93.9019) -> (-61.5684, -93.1668) centre (-101.8395, -75.4579) ccw
  arc A373 (-61.5684, -93.1668) -> (-61.7798, -92.4963) centre (-62.0567, -92.9521) ccw
  arc A374 (-62.3466, -92.0385) -> (-61.7798, -92.4963) centre (-60.3577, -90.1556) ccw
  arc A375 (-61.4197, -89.6297) -> (-62.3466, -92.0385) centre (-61.3082, -91.0553) ccw
  arc A376 (-60.6921, -89.67) -> (-61.4197, -89.6297) centre (-61.2061, -92.3602) ccw
  arc A377 (-60.6921, -89.67) -> (-60.0858, -89.3141) centre (-60.5921, -89.1461) ccw
  arc A378 (-60.0858, -89.3141) -> (-59.8389, -88.5466) centre (-101.8395, -75.4579) ccw
  arc A379 (-59.8389, -88.5466) -> (-60.124, -87.9039) centre (-60.3481, -88.3879) ccw
  arc A380 (-60.7385, -87.5124) -> (-60.124, -87.9039) centre (-58.9729, -85.4187) ccw
  arc A381 (-60.0871, -85.015) -> (-60.7385, -87.5124) centre (-59.8167, -86.4192) ccw
  arc A382 (-59.3596, -84.9736) -> (-60.0871, -85.015) centre (-59.5691, -87.7044) ccw
  arc A383 (-59.3596, -84.9736) -> (-58.7969, -84.552) centre (-59.3188, -84.4417) ccw
  arc A384 (-58.7969, -84.552) -> (-58.6375, -83.7617) centre (-101.8395, -75.4579) ccw
  arc A385 (-58.6375, -83.7617) -> (-58.9928, -83.1549) centre (-59.1613, -83.661) ccw
  arc A386 (-59.6473, -82.8348) -> (-58.9928, -83.1549) centre (-58.1272, -80.5565) ccw
  arc A387 (-59.2796, -80.2801) -> (-59.6473, -82.8348) centre (-58.8536, -81.6452) ccw
  arc A388 (-58.5613, -80.1575) -> (-59.2796, -80.2801) centre (-58.4638, -82.8946) ccw
  arc A389 (-58.5613, -80.1575) -> (-58.0494, -79.6756) centre (-58.5803, -79.6244) ccw
  arc A390 (-58.0494, -79.6756) -> (-57.9794, -78.8724) centre (-101.8395, -75.4579) ccw
  arc A391 (-57.9794, -78.8724) -> (-58.4004, -78.3092) centre (-58.5112, -78.831) ccw
  arc A392 (-59.0867, -78.0643) -> (-58.4004, -78.3092) centre (-57.8312, -75.6302) ccw
  arc A393 (-59.0073, -75.4846) -> (-59.0867, -78.0643) centre (-58.4312, -76.7934) ccw
  arc A394 (-58.3073, -75.2823) -> (-59.0073, -75.4846) centre (-57.9039, -77.9913) ccw
  arc A395 (-58.3073, -75.2823) -> (-57.8525, -74.7461) centre (-58.3858, -74.7547) ccw
  arc A396 (-57.8525, -74.7461) -> (-57.8729, -73.9401) centre (-101.8395, -75.4579) ccw
  arc A397 (-57.8729, -73.9401) -> (-58.3543, -73.4277) centre (-58.406, -73.9585) ccw
  arc A398 (-59.0637, -73.2611) -> (-58.3543, -73.4277) centre (-58.0887, -70.7017) ccw
  arc A399 (-59.2736, -70.6887) -> (-59.0637, -73.2611) centre (-58.5546, -71.9248) ccw
  arc A400 (-58.6006, -70.4094) -> (-59.2736, -70.6887) centre (-57.8965, -73.0561) ccw
  arc A401 (-58.6006, -70.4094) -> (-58.2088, -69.8256) centre (-58.7378, -69.8939) ccw
  arc A402 (-58.2088, -69.8256) -> (-58.3193, -69.027) centre (-101.8395, -75.4579) ccw
  arc A403 (-58.3193, -69.027) -> (-58.855, -68.5716) centre (-58.847, -69.105) ccw
  arc A404 (-59.5786, -68.4856) -> (-58.855, -68.5716) centre (-58.8963, -65.8331) ccw
  arc A405 (-60.0753, -65.9528) -> (-59.5786, -68.4856) centre (-59.2223, -67.1006) ccw
  arc A406 (-59.4378, -65.5999) -> (-60.0753, -65.9528) centre (-58.4417, -68.1512) ccw
  arc A407 (-59.4378, -65.5999) -> (-59.1137, -64.9759) centre (-59.6318, -65.103) ccw
  arc A408 (-59.1137, -64.9759) -> (-59.313, -64.1947) centre (-101.8395, -75.4579) ccw
  arc A409 (-59.313, -64.1947) -> (-59.8963, -63.8022) centre (-59.8286, -64.3313) ccw
  arc A410 (-60.625, -63.7977) -> (-59.8963, -63.8022) centre (-60.2439, -61.0855) ccw
  arc A411 (-61.4021, -61.3365) -> (-60.625, -63.7977) centre (-60.426, -62.3816) ccw
  arc A412 (-60.8081, -60.9144) -> (-61.4021, -61.3365) centre (-59.5327, -63.3381) ccw
  arc A413 (-60.8081, -60.9144) -> (-60.556, -60.2581) centre (-61.0566, -60.4424) ccw
  arc A414 (-60.556, -60.2581) -> (-60.8415, -59.5041) centre (-101.8395, -75.4579) ccw
  arc A415 (-60.8415, -59.5041) -> (-61.4651, -59.1793) centre (-61.3386, -59.6975) ccw
  arc A416 (-62.1896, -59.2564) -> (-61.4651, -59.1793) centre (-62.1147, -56.5186) ccw
  arc A417 (-63.2375, -56.8977) -> (-62.1896, -59.2564) centre (-62.1505, -57.827) ccw
  arc A418 (-62.6945, -56.4118) -> (-63.2375, -56.8977) centre (-61.1557, -58.6774) ccw
  arc A419 (-62.6945, -56.4118) -> (-62.5174, -55.7313) centre (-62.9942, -55.9705) ccw
  arc A420 (-62.5174, -55.7313) -> (-62.8855, -55.0141) centre (-101.8395, -75.4579) ccw
  arc A421 (-62.8855, -55.0141) -> (-63.5416, -54.7612) centre (-63.3578, -55.2619) ccw
  arc A422 (-64.253, -54.9189) -> (-63.5416, -54.7612) centre (-64.485, -52.19) ccw
  arc A423 (-65.5583, -52.6924) -> (-64.253, -54.9189) centre (-64.3741, -53.4941) ccw
  arc A424 (-65.0731, -52.1487) -> (-65.5583, -52.6924) centre (-63.2903, -54.2278) ccw
  arc A425 (-65.0731, -52.1487) -> (-64.9734, -51.4527) centre (-65.4203, -51.7438) ccw
  arc A426 (-64.9734, -51.4527) -> (-65.4195, -50.7811) centre (-101.8395, -75.4579) ccw
  arc A427 (-65.4195, -50.7811) -> (-66.0997, -50.6033) centre (-65.861, -51.0803) ccw
  arc A428 (-66.7889, -50.8397) -> (-66.0997, -50.6033) centre (-67.3251, -48.1539) ccw
  arc A429 (-68.3353, -48.7733) -> (-66.7889, -50.8397) centre (-67.0689, -49.4374) ccw
  arc A430 (-67.9141, -48.1787) -> (-68.3353, -48.7733) centre (-65.9097, -50.0451) ccw
  arc A431 (-67.9141, -48.1787) -> (-67.8929, -47.4759) centre (-68.3045, -47.8152) ccw
  arc A432 (-67.8929, -47.4759) -> (-68.4114, -46.8585) centre (-101.8395, -75.4579) ccw
  arc A433 (-68.4114, -46.8585) -> (-69.1073, -46.758) centre (-68.8167, -47.2053) ccw
  arc A434 (-69.7657, -47.0701) -> (-69.1073, -46.758) centre (-70.5992, -44.4612) ccw
  arc A435 (-71.5337, -45.1898) -> (-69.7657, -47.0701) centre (-70.2009, -45.7079) ccw
  arc A436 (-71.1817, -44.5518) -> (-71.5337, -45.1898) centre (-68.981, -46.1821) ccw
  arc A437 (-71.1817, -44.5518) -> (-71.2393, -43.8511) centre (-71.6104, -44.2343) ccw
  arc A438 (-71.2393, -43.8511) -> (-71.8237, -43.2956) centre (-101.8395, -75.4579) ccw
  arc A439 (-71.8237, -43.2956) -> (-72.5264, -43.2736) centre (-72.1876, -43.6856) ccw
  arc A440 (-73.1458, -43.6575) -> (-72.5264, -43.2736) centre (-74.2661, -41.1583) ccw
  arc A441 (-75.1132, -41.9869) -> (-73.1458, -43.6575) centre (-73.7308, -42.3525) ccw
  arc A442 (-74.8349, -41.3135) -> (-75.1132, -41.9869) centre (-72.4654, -42.6872) ccw
  arc A443 (-74.8349, -41.3135) -> (-74.9706, -40.6237) centre (-75.2964, -41.046) ccw
  arc A444 (-74.9706, -40.6237) -> (-75.6135, -40.1371) centre (-101.8395, -75.4579) ccw
  arc A445 (-75.6135, -40.1371) -> (-76.3143, -40.1939) centre (-75.9315, -40.5654) ccw
  arc A446 (-76.8867, -40.6447) -> (-76.3143, -40.1939) centre (-78.2798, -38.2867) ccw
  arc A447 (-79.0289, -39.205) -> (-76.8867, -40.6447) centre (-77.6141, -39.4135) ccw
  arc A448 (-78.8277, -38.5047) -> (-79.0289, -39.205) centre (-76.3193, -39.6044) ccw
  arc A449 (-78.8277, -38.5047) -> (-79.0397, -37.8343) centre (-79.3162, -38.2905) ccw
  arc A450 (-79.0397, -37.8343) -> (-79.7331, -37.4228) centre (-101.8395, -75.4579) ccw
  arc A451 (-79.7331, -37.4228) -> (-80.4231, -37.5577) centre (-80.0011, -37.884) ccw
  arc A452 (-80.9415, -38.0698) -> (-80.4231, -37.5577) centre (-82.5898, -35.8826) ccw
  arc A453 (-83.2313, -36.879) -> (-80.9415, -38.0698) centre (-81.8021, -36.9278) ccw
  arc A454 (-83.1098, -36.1605) -> (-83.2313, -36.879) centre (-80.4941, -36.9724) ccw
  arc A455 (-83.1098, -36.1605) -> (-83.3956, -35.5181) centre (-83.6192, -36.0024) ccw
  arc A456 (-83.3956, -35.5181) -> (-84.1306, -35.1868) centre (-101.8395, -75.4579) ccw
  line L37 (-121.8728, 32.134) -> (-90.1228, 6.734)
  line L38 (-121.8728, 6.734) -> (-90.1228, 32.134)
  circle A457 centre (-171.542, -73.2557) radius 14.2748
  circle A458 centre (-105.9978, 19.434) radius 21.4859
  circle A459 centre (-171.542, -73.2557) radius 14.3243
  line L39 (-160.3914, -82.2474) -> (-89.2724, 5.9468)
  line L40 (-124.2883, 30.7078) -> (-183.736, -65.7396)
  line L41 (-193.767, -95.4807) -> (-149.317, -95.4807)
  line L42 (-149.317, -95.4807) -> (-149.317, -51.0307)
  line L43 (-149.317, -51.0307) -> (-193.767, -51.0307)
  line L44 (-193.767, -51.0307) -> (-193.767, -95.4807)
  line L45 (-193.767, -95.4807) -> (-149.317, -51.0307) construction
  line L46 (-149.317, -95.4807) -> (-193.767, -51.0307) construction
  circle A460 centre (-171.542, -73.2557) radius 31.4309
  arc A461 (-181.9312, -110.8876) -> (-185.6678, -111.3086) centre (-183.1204, -117.1252) ccw
  arc A462 (-174.8852, -173.4224) -> (-181.9312, -110.8876) centre (-180.2765, -142.3655) ccw
  arc A463 (-178.6218, -173.8435) -> (-174.8852, -173.4224) centre (-177.4326, -167.6058) ccw
  arc A464 (-185.6678, -111.3086) -> (-178.6218, -173.8435) centre (-180.2765, -142.3655) ccw
  arc A465 (-181.7907, -98.8592) -> (-182.3406, -98.4212) centre (-182.3156, -98.954) ccw
  arc A466 (-182.3406, -98.4212) -> (-183.1456, -98.4664) centre (-180.2765, -142.3655) ccw
  arc A467 (-183.1456, -98.4664) -> (-183.643, -98.9632) centre (-183.1108, -98.9986) ccw
  arc A468 (-183.7876, -99.6774) -> (-183.643, -98.9632) centre (-186.3758, -98.7816) ccw
  arc A469 (-186.3524, -99.9664) -> (-183.7876, -99.6774) centre (-185.139, -99.2097) ccw
  arc A470 (-186.6523, -99.3023) -> (-186.3524, -99.9664) centre (-184.0285, -98.5171) ccw
  arc A471 (-186.6523, -99.3023) -> (-187.2478, -98.9286) centre (-187.1633, -99.4552) ccw
  arc A472 (-187.2478, -98.9286) -> (-188.0427, -99.0636) centre (-180.2765, -142.3655) ccw
  arc A473 (-188.0427, -99.0636) -> (-188.4814, -99.6131) centre (-187.9485, -99.5887) ccw
  arc A474 (-188.5451, -100.3389) -> (-188.4814, -99.6131) centre (-191.2173, -99.7385) ccw
  arc A475 (-191.0614, -100.9133) -> (-188.5451, -100.3389) centre (-189.9403, -100.0254) ccw
  arc A476 (-191.4338, -100.2869) -> (-191.0614, -100.9133) centre (-188.9143, -99.2129) ccw
  arc A477 (-191.4338, -100.2869) -> (-192.0674, -99.9822) centre (-191.9244, -100.4961) ccw
  arc A478 (-192.0674, -99.9822) -> (-192.8421, -100.2054) centre (-180.2765, -142.3655) ccw
  arc A479 (-192.8421, -100.2054) -> (-193.2165, -100.8006) centre (-192.6898, -100.7166) ccw
  arc A480 (-193.1986, -101.529) -> (-193.2165, -100.8006) centre (-195.9212, -101.2315) ccw
  arc A481 (-195.6348, -102.3814) -> (-193.1986, -101.529) centre (-194.6202, -101.3737) ccw
  arc A482 (-196.0749, -101.8007) -> (-195.6348, -102.3814) centre (-193.6916, -100.4513) ccw
  arc A483 (-196.0749, -101.8007) -> (-196.7387, -101.5689) centre (-196.5391, -102.0636) ccw
  arc A484 (-196.7387, -101.5689) -> (-197.4835, -101.8774) centre (-180.2765, -142.3655) ccw
  arc A485 (-197.4835, -101.8774) -> (-197.789, -102.5107) centre (-197.2749, -102.3683) ccw
  arc A486 (-197.6896, -103.2326) -> (-197.789, -102.5107) centre (-200.4284, -103.2418) ccw
  arc A487 (-200.015, -104.3524) -> (-197.6896, -103.2326) centre (-199.1196, -103.2374) ccw
  arc A488 (-200.5174, -103.8247) -> (-200.015, -104.3524) centre (-198.3001, -102.2169) ccw
  arc A489 (-200.5174, -103.8247) -> (-201.2029, -103.6686) centre (-200.9492, -104.1378) ccw
  arc A490 (-201.2029, -103.6686) -> (-201.9086, -104.0586) centre (-180.2765, -142.3655) ccw
  arc A491 (-201.9086, -104.0586) -> (-202.1412, -104.7221) centre (-201.6463, -104.5231) ccw
  arc A492 (-201.9616, -105.4283) -> (-202.1412, -104.7221) centre (-204.6822, -105.7441) ccw
  arc A493 (-204.147, -106.8014) -> (-201.9616, -105.4283) centre (-203.3821, -105.5932) ccw
  arc A494 (-204.7053, -106.3333) -> (-204.147, -106.8014) centre (-202.682, -104.4874) ccw
  arc A495 (-204.7053, -106.3333) -> (-205.404, -106.2549) centre (-205.0994, -106.6928) ccw
  arc A496 (-205.404, -106.2549) -> (-206.0616, -106.7215) centre (-180.2765, -142.3655) ccw
  arc A497 (-206.0616, -106.7215) -> (-206.2184, -107.4069) centre (-205.7489, -107.1537) ccw
  arc A498 (-205.9609, -108.0885) -> (-206.2184, -107.4069) centre (-208.629, -108.707) ccw
  arc A499 (-207.9788, -109.6977) -> (-205.9609, -108.0885) centre (-207.354, -108.4114) ccw
  arc A500 (-208.5861, -109.295) -> (-207.9788, -109.6977) centre (-206.7821, -107.2342) ccw
  arc A501 (-208.5861, -109.295) -> (-209.2891, -109.2954) centre (-208.9374, -109.6964) ccw
  arc A502 (-209.2891, -109.2954) -> (-209.8903, -109.8326) centre (-180.2765, -142.3655) ccw
  arc A503 (-209.8903, -109.8326) -> (-209.9694, -110.5312) centre (-209.5312, -110.2271) ccw
  arc A504 (-209.6372, -111.1798) -> (-209.9694, -110.5312) centre (-212.2193, -112.0931) ccw
  arc A505 (-211.4623, -113.0048) -> (-209.6372, -111.1798) centre (-210.9854, -111.6566) ccw
  arc A506 (-212.1108, -112.6726) -> (-211.4623, -113.0048) centre (-210.5489, -110.4227) ccw
  arc A507 (-212.1108, -112.6726) -> (-212.8094, -112.7517) centre (-212.4149, -113.1108) ccw
  arc A508 (-212.8094, -112.7517) -> (-213.3466, -113.3529) centre (-180.2765, -142.3655) ccw
  arc A509 (-213.3466, -113.3529) -> (-213.347, -114.056) centre (-212.9457, -113.7046) ccw
  arc A510 (-212.9443, -114.6632) -> (-213.347, -114.056) centre (-215.4079, -115.8599) ccw
  arc A511 (-214.5535, -116.6811) -> (-212.9443, -114.6632) centre (-214.2306, -115.288) ccw
  arc A512 (-215.2352, -116.4236) -> (-214.5535, -116.6811) centre (-213.9351, -114.013) ccw
  arc A513 (-215.2352, -116.4236) -> (-215.9205, -116.5804) centre (-215.4884, -116.8931) ccw
  arc A514 (-215.9205, -116.5804) -> (-216.3871, -117.238) centre (-180.2765, -142.3655) ccw
  arc A515 (-216.3871, -117.238) -> (-216.3087, -117.9367) centre (-215.9492, -117.5426) ccw
  arc A516 (-215.8406, -118.495) -> (-216.3087, -117.9367) centre (-218.1547, -119.96) ccw
  arc A517 (-217.2137, -120.6804) -> (-215.8406, -118.495) centre (-217.0488, -119.2599) ccw
  arc A518 (-217.9199, -120.5008) -> (-217.2137, -120.6804) centre (-216.8979, -117.9599) ccw
  arc A519 (-217.9199, -120.5008) -> (-218.5834, -120.7334) centre (-218.119, -120.9957) ccw
  arc A520 (-218.5834, -120.7334) -> (-218.9734, -121.4391) centre (-180.2765, -142.3655) ccw
  arc A521 (-218.9734, -121.4391) -> (-218.8173, -122.1246) centre (-218.5042, -121.6928) ccw
  arc A522 (-218.2896, -122.627) -> (-218.8173, -122.1246) centre (-220.4251, -124.3419) ccw
  arc A523 (-219.4094, -124.9524) -> (-218.2896, -122.627) centre (-219.4046, -123.5224) ccw
  arc A524 (-220.1313, -124.8531) -> (-219.4094, -124.9524) centre (-219.4002, -122.2136) ccw
  arc A525 (-220.1313, -124.8531) -> (-220.7646, -125.1585) centre (-220.2737, -125.3671) ccw
  arc A526 (-220.7646, -125.1585) -> (-221.0731, -125.9033) centre (-180.2765, -142.3655) ccw
  arc A527 (-221.0731, -125.9033) -> (-220.8413, -126.5671) centre (-220.5785, -126.1029) ccw
  arc A528 (-220.2606, -127.0073) -> (-220.8413, -126.5671) centre (-222.1907, -128.9504) ccw
  arc A529 (-221.113, -129.4434) -> (-220.2606, -127.0073) centre (-221.2683, -128.0218) ccw
  arc A530 (-221.8415, -129.4255) -> (-221.113, -129.4434) centre (-221.4105, -126.7208) ccw
  arc A531 (-221.8415, -129.4255) -> (-222.4366, -129.7999) centre (-221.9254, -129.9522) ccw
  arc A532 (-222.4366, -129.7999) -> (-222.6598, -130.5746) centre (-180.2765, -142.3655) ccw
  arc A533 (-222.6598, -130.5746) -> (-222.3551, -131.2083) centre (-222.1459, -130.7176) ccw
  arc A534 (-221.7287, -131.5806) -> (-222.3551, -131.2083) centre (-223.4291, -133.7277) ccw
  arc A535 (-222.3031, -134.0969) -> (-221.7287, -131.5806) centre (-222.6166, -132.7017) ccw
  arc A536 (-223.0289, -134.1607) -> (-222.3031, -134.0969) centre (-222.9035, -131.4247) ccw
  arc A537 (-223.0289, -134.1607) -> (-223.5784, -134.5993) centre (-223.0534, -134.6935) ccw
  arc A538 (-223.5784, -134.5993) -> (-223.7134, -135.3942) centre (-180.2765, -142.3655) ccw
  arc A539 (-223.7134, -135.3942) -> (-223.3397, -135.9897) centre (-223.1868, -135.4787) ccw
  arc A540 (-222.6756, -136.2896) -> (-223.3397, -135.9897) centre (-224.1249, -138.6136) ccw
  arc A541 (-222.9646, -138.8544) -> (-222.6756, -136.2896) centre (-223.4324, -137.503) ccw
  arc A542 (-223.6788, -138.999) -> (-222.9646, -138.8544) centre (-223.8604, -136.2662) ccw
  arc A543 (-223.6788, -138.999) -> (-224.1756, -139.4964) centre (-223.6434, -139.5312) ccw
  arc A544 (-224.1756, -139.4964) -> (-224.2209, -140.3014) centre (-180.2765, -142.3655) ccw
  arc A545 (-224.2209, -140.3014) -> (-223.7828, -140.8513) centre (-223.688, -140.3264) ccw
  arc A546 (-223.0893, -141.075) -> (-223.7828, -140.8513) centre (-224.2693, -143.5466) ccw
  arc A547 (-223.0893, -143.656) -> (-223.0893, -141.075) centre (-223.7054, -142.3655) ccw
  arc A548 (-223.7828, -143.8797) -> (-223.0893, -143.656) centre (-224.2693, -141.1844) ccw
  arc A549 (-223.7828, -143.8797) -> (-224.2209, -144.4296) centre (-223.688, -144.4046) ccw
  arc A550 (-224.2209, -144.4296) -> (-224.1756, -145.2346) centre (-180.2765, -142.3655) ccw